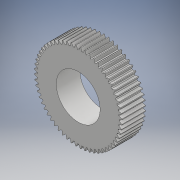
# Autodesk Inventor part: Шестерня 2
Saved by Autodesk Inventor 2018.1 (Build 221171000, 171)
## iProperties
Created: 2018-06-08
Part Number: Шестерня 2
Material: Типовые
Document SubType Name: Modeling
Designer: Dmitry
Density: 1 g/cm^3
Appearance: По умолчанию
Author: Dmitry
Autodesk Inventor part; units mm, degrees
ref_plane "YZ Plane" through (0, 0, 0) normal (1, 0, 0) x (0, 1, 0)
ref_plane "XZ Plane" through (0, 0, 0) normal (0, 1, 0) x (-1, 0, 0)
ref_plane "XY Plane" through (0, 0, 0) normal (0, 0, 1) x (1, 0, 0)
sketch "Эскиз1" plane through (0, 0, 0) normal (0, 0, 1) x (1, 0, 0)
  line L0 (31, 0) -> (62, 0)
  line L1 (62, 0) -> (62, 33.3333)
  line L2 (62, 33.3333) -> (31, 33.3333)
  line L3 (31, 33.3333) -> (31, 0)
  line L4 (0, -6.6667) -> (0, 40) projected
  constraints: 8 end point
revolve "Вращение1" add sketch "Эскиз1" angle 360 about axis through (0, -10, 0) along (0, 1, 0)
sketch "Эскиз2" plane through (0, 0, 0) normal (0, 1, 0) x (-1, 0, 0)
  line L0 (2.7475, 61.9391) -> (0.785, 57.6846)
  line L1 (-2.7475, 61.9391) -> (-0.785, 57.6846)
  arc A0 (2.7475, 61.9391) -> (-2.7475, 61.9391) centre (0, 0) ccw
  arc A1 (0.785, 57.6846) -> (-0.785, 57.6846) centre (0, 53.0057) ccw
  constraints: 4 end point, 4 point on circle, 2 centre point
extrude "Выдавливание1" cut sketch "Эскиз2" along normal blind 33.3333
pattern_circular "Круговой массив1" count 60 over 360 about axis through (0, -10, 0) along (0, 1, 0) of "Выдавливание1"
